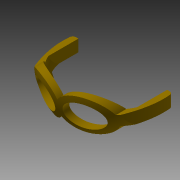
# Autodesk Inventor part: Ojo
Saved by Autodesk Inventor 2014 (Build 180170000, 170)
## iProperties
Created: 2015-01-03
Part Number: Ojo
Material: Generic
Document SubType Name: Modeling
Designer: Rubén
Density: 1 g/cm^3
Appearance: Gold
d0: 15,000 mm
d5: 17,000 mm
Author: Rubén
Autodesk Inventor part; units mm, degrees
sketch "Sketch2" plane through (0, 0, 0) normal (0, 1, 0) x (-1, 0, 0)
  arc A0 (15, 0) -> (-15, 0) centre (0, 0) ccw
  line L0 (-15, 0) -> (15, 0)
  dimension "d0" = 15
  constraints: 2 end point, 2 point on circle, 1 centre point, 1 coincident, 1 horizontal
  measures "d0" radius of A0
sketch "Sketch5" plane through (0, 0, 0) normal (0, 0, 1) x (1, 0, 0)
  ellipse E0 centre (-6, -4) end of major axis (-1.2, -4) minor radius 3.8
  ellipse E1 centre (-6, -4) end of major axis (0.7, -4) minor radius 5.5 (-12.331, -5.8) -> (-12.331, -2.2) ccw
  line L0 (-12.331, -2.2) -> (-32.331, -2.2)
  line L1 (-32.331, -2.2) -> (-32.331, -5.8)
  line L2 (-32.331, -5.8) -> (-12.331, -5.8)
  line L3 (0, 3.3285) -> (0, -12.076) construction
  ellipse E2 centre (6, -4) end of major axis (1.2, -4) minor radius 3.8
  ellipse E3 centre (6, -4) end of major axis (-0.7, -4) minor radius 5.5 (12.331, -2.2) -> (12.331, -5.8) ccw
  line L4 (12.331, -2.2) -> (32.331, -2.2)
  line L5 (32.331, -2.2) -> (32.331, -5.8)
  line L6 (32.331, -5.8) -> (12.331, -5.8)
  point P0 (0, 0)
  point P1 (-1.2, -4)
  point P2 (0.7, -4)
  point P3 (-6, 1.5)
  dimension "d19" = 3.8
  dimension "d20" = 4.8
  dimension "d17" = 6
  dimension "d18" = 4
  dimension "d27" = 20
  dimension "d28" = 3.6
  constraints: 14 end point, 7 symmetric about line, 4 vertical, 3 coincident, 2 point on line, 1 horizontal, 1 horizontal alignment, 14 other
  measures "d17" horizontal distance of point (-6, -4) point (0, 0)
  measures "d18" vertical distance of point (-6, -4) point (0, 0)
  measures "d27" distance of L0.start L0.end
  measures "d28" distance of L0.end L1.end
sketch "Sketch6" plane through (0, 0, 0) normal (0, 1, 0) x (-1, 0, 0)
  arc A0 (17, 0) -> (-17, 0) centre (0, 0) ccw
  line L0 (-17, 0) -> (17, 0)
  dimension "d5" = 17
  constraints: 2 end point, 2 point on circle, 1 centre point, 1 coincident, 1 horizontal
  measures "d5" radius of A0
ref_plane "Work Plane1" through (0, 0, 0) normal (-1, 0, 0) x (0, -1, 0)
sketch "Sketch8" plane through (0, 0, 0) normal (-1, 0, 0) x (0, -1, 0)
  line L0 (-3, -10) -> (-3, 20)
  line L1 (-3, 20) -> (15, 20)
  line L2 (15, 20) -> (15, -10)
  line L3 (15, -10) -> (-3, -10)
  point P0 (0, 0)
  dimension "d21" = 30
  dimension "d22" = 18
  dimension "d29" = 3
  dimension "d30" = 20
  constraints: 8 end point, 2 parallel, 1 perpendicular, 1 vertical
  measures "d21" distance of L0.start L0.end
  measures "d22" distance of L0.end L1.end
  measures "d29" distance from line of L0 point (0, 0)
  measures "d30" distance from line of L1 point (0, 0)
extrude "Extrusion4" add sketch "Sketch8" along normal mid plane 40
revolve "Revolution1" cut sketch "Sketch2" angle 360 about axis through (15, 0, 0) along (-1, 0, 0)
revolve "Revolution2" cut sketch "Sketch6" angle 360 about axis through (17, 0, 0) along (-1, 0, 0) keep common part
extrude "Extrusion5" cut sketch "Sketch5" along normal blind 20 and the other way blind 3 keep common part
ref_plane "Work Plane3" through (15.6959, -5.8, -3) normal (0, 0, -1) x (-1, 0, 0)
sketch "Sketch10" plane through (15.6959, -5.8, -3) normal (0, 0, -1) x (-1, 0, 0)
  line L0 (2.1959, 7.5076) -> (2.1959, -4.0049) construction
  line L1 (2.1959, 0) -> (0.566, 0)
  line L2 (0.566, 0) -> (0.566, 3.6)
  line L3 (0.566, 3.6) -> (2.1959, 3.6)
  line L4 (2.1959, 3.6) -> (2.1959, 0)
  line L5 (15.6959, 5.8) -> (15.6959, -2.5433) construction
  line L6 (29.1959, 0) -> (30.8257, 0)
  line L7 (30.8257, 0) -> (30.8257, 3.6)
  line L8 (30.8257, 3.6) -> (29.1959, 3.6)
  line L9 (29.1959, 3.6) -> (29.1959, 0)
  dimension "d33" = 13.5
  dimension "d34" = 3.6
  constraints: 20 end point, 4 symmetric about line, 3 parallel, 1 horizontal, 1 perpendicular, 1 point on line, 1 vertical
  measures "d33" distance from line of L0 L5.start
  measures "d34" distance of L1.end L2.end
extrude "Extrusion6" add sketch "Sketch10" against normal up to next
ref_plane "Work Plane4" through (-13.5, -5.8, -3) normal (0, -1, 0) x (1, 0, 0)
sketch "Sketch13" plane through (-13.5, -5.8, -3) normal (0, -1, 0) x (1, 0, 0)
  line L0 (-1.6339, -0.0649) -> (-1.9763, 2.5198) construction
  line L1 (-1.9763, 2.5198) -> (-1.9763, 5.3741) construction
  line L2 (-1.9763, 5.3741) -> (-1.3834, 9.037) construction
  line L3 (-1.3834, 9.037) -> (0.471, 13.7458) construction
  spline S0 degree 4 poles (-1.6339, -0.0649) (-1.9763, 2.5198) (-1.9763, 5.3741) (-1.3834, 9.037) (0.471, 13.7458) knots 1 1 1 1 1 2 2 2 2 2
  line L4 (0.471, 13.7458) -> (-3.7388, 13.7458)
  line L5 (-3.7388, 13.7458) -> (-3.7388, -0.0649)
  line L6 (-3.7388, -0.0649) -> (-1.6339, -0.0649)
  line L7 (13.5, 3) -> (13.5, 11.3386) construction
  line L8 (28.6339, -0.0649) -> (28.9763, 2.5198) construction
  line L9 (28.9763, 2.5198) -> (28.9763, 5.3741) construction
  line L10 (28.9763, 5.3741) -> (28.3834, 9.037) construction
  line L11 (28.3834, 9.037) -> (26.529, 13.7458) construction
  spline S1 degree 4 poles (28.6339, -0.0649) (28.9763, 2.5198) (28.9763, 5.3741) (28.3834, 9.037) (26.529, 13.7458) knots 1 1 1 1 1 2 2 2 2 2
  line L12 (26.529, 13.7458) -> (30.7388, 13.7458)
  line L13 (30.7388, 13.7458) -> (30.7388, -0.0649)
  line L14 (30.7388, -0.0649) -> (28.6339, -0.0649)
  constraints: 14 end point, 7 symmetric about line, 3 perpendicular, 1 parallel, 6 other
extrude "Extrusion8" cut sketch "Sketch13" against normal through all
fillet "Fillet2" radius 1 2 edges at (15.1424, -3.9832, -3) (-15.1424, -3.9832, -3)
body "Solid1"
